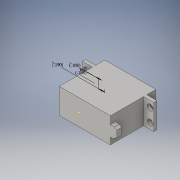
# Autodesk Inventor part: Aidan Sherry Servo motor
Saved by Autodesk Inventor 2016 (Build 200138000, 138)
## iProperties
Created: 2016-10-05
Part Number: Aidan Sherry Servo motor
Material: Generic
Document SubType Name: Modeling
Designer: sherra
Density: 1 g/cm^3
Appearance: Default
Author: sherra
Autodesk Inventor part; units mm, degrees
ref_plane "YZ Plane" through (0, 0, 0) normal (1, 0, 0) x (0, 1, 0)
ref_plane "XZ Plane" through (0, 0, 0) normal (0, 1, 0) x (-1, 0, 0)
ref_plane "XY Plane" through (0, 0, 0) normal (0, 0, 1) x (1, 0, 0)
sketch "Sketch1" plane through (0, 0, 0) normal (0, 0, 1) x (1, 0, 0)
  line L0 (-15.561, 10.0244) -> (24.939, 10.0244)
  line L1 (24.939, 10.0244) -> (24.939, -9.9756)
  line L2 (24.939, -9.9756) -> (-15.561, -9.9756)
  line L3 (-15.561, -9.9756) -> (-15.561, 10.0244)
  point P0 (0, 0)
  dimension "d0" = 20
  dimension "d1" = 40.5
  constraints: 8 end point, 2 parallel, 1 horizontal, 1 perpendicular
  measures "d0" distance between parallel lines of L2 L0
  measures "d1" distance of L0.start L0.end
extrude "Extrusion1" add sketch "Sketch1" along normal blind 36.1
sketch "Sketch2" plane through (24.939, -9.9756, 0) normal (1, 0, 0) x (0, 0, -1)
  line L0 (-36.1, 20) -> (-36.1, 0) projected
  line L1 (-36.1, 13.8904) -> (-32.1201, 13.8904)
  line L2 (-32.1201, 13.8904) -> (-32.1201, 5.486)
  line L3 (-32.1201, 5.486) -> (-36.1, 5.486)
  line L4 (-36.1, 5.486) -> (-36.1, 13.8904)
  point P0 (0, 9.9756)
  constraints: 8 end point, 2 parallel, 1 horizontal, 1 perpendicular, 1 point on line
extrude "Extrusion2" add sketch "Sketch2" along normal blind 5.08
sketch "Sketch3" plane through (24.939, -9.9756, 0) normal (1, 0, 0) x (0, 0, -1)
  line L0 (-36.1, 13.8904) -> (-36.1, 20) projected
  line L1 (-7.2964, 16.9452) -> (-7.2964, 3.5991)
  line L2 (-9.7348, 3.5991) -> (-9.7348, 16.9452)
  line L3 (-9.7348, 16.9452) -> (-9.7348, 20)
  line L4 (0, 20) -> (-36.1, 20) projected
  line L5 (-7.2964, 16.9452) -> (-7.2964, 20)
  line L6 (-7.2964, 3.5991) -> (-7.2964, 0)
  line L7 (0, 0) -> (-36.1, 0) projected
  line L8 (-9.7348, 3.5991) -> (-9.7348, 0)
  point P0 (0, 9.9756)
  constraints: 12 end point, 6 point on line, 2 parallel, 1 vertical
extrude "Extrusion3" add sketch "Sketch3" along normal blind 8.0264
sketch "Sketch4" plane through (-15.561, -9.9756, 0) normal (-1, 0, 0) x (0, 0, 1)
  line L0 (0, 0) -> (7.2964, 0) projected
  line L1 (9.7348, 20) -> (36.1, 20) projected
  line L2 (7.2964, 0) -> (9.7348, 0)
  line L3 (9.7348, 0) -> (9.7348, 20)
  line L4 (9.7348, 20) -> (7.2964, 20)
  line L5 (7.2964, 20) -> (7.2964, 0)
  point P0 (0, 9.9756)
  constraints: 8 end point, 2 parallel, 1 horizontal, 1 perpendicular
extrude "Extrusion4" add sketch "Sketch4" along normal blind 8.0264
sketch "Sketch5" plane through (24.939, -9.9756, 7.2964) normal (0, 0, -1) x (-1, 0, 0)
  line L0 (0, 20) -> (-8.0264, 20) projected
  circle A0 centre (-5.1734, 4.773) radius 2.3347
  line L1 (40.5, 0) -> (48.5264, 0) projected
  line L2 (40.5, 20) -> (48.5264, 20) projected
  circle A1 centre (45.3266, 4.773) radius 2.3347
  circle A2 centre (45.3266, 15.1496) radius 2.3347
  circle A3 centre (-5.1734, 15.1496) radius 2.3347
  point P0 (24.939, 9.9756)
  dimension "d18" = 50.5
  constraints: 4 centre point
  measures "d18" distance of A2.centre A3.centre
hole "Hole1" at (30.1124, -5.2026, 7.2964) at (30.1124, 5.174, 7.2964) at (-20.3876, -5.2026, 7.2964) at (-20.3876, 5.174, 7.2964) direction (0, 0, 1) diameter 4.7625 end through all
sketch "Sketch6" plane through (0, 0, 0) normal (0, 0, -1) x (-1, 0, 0)
  line L0 (15.561, -9.9756) -> (15.561, 10.0244) projected
  line L1 (15.561, 0.0244) -> (-14.839, 0.0244)
  circle A0 centre (-14.839, 0.0244) radius 2.9972
  point P0 (0, 0)
  dimension "d26" = 30.4
  dimension "d27" = 5.9944
  constraints: 2 end point, 1 centre point, 1 coincident, 1 horizontal, 1 midpoint
  measures "d26" distance of L1.start L1.end
  measures "d27" diameter of A0
extrude "Extrusion5" add sketch "Sketch6" along normal blind 5.9944
sketch "Sketch7" plane through (0, 0, 36.1) normal (0, 0, 1) x (1, 0, 0)
  point P0 (0, 0)
sketch "Sketch8" plane through (0, 0, 0) normal (0, 0, -1) x (-1, 0, 0)
  line L0 (15.561, -9.9756) -> (15.561, 10.0244) projected
  circle A0 centre (20.3876, -5.2026) radius 2.3813 projected
  line L1 (15.561, -9.9756) -> (23.5874, -9.9756) projected
  point P0 (0, 0)
  dimension "d30" = 4.8266
  dimension "d31" = 4.7625
  dimension "d33" = 4.773
  measures "d30" distance from line of L0 A0.centre
  measures "d31" diameter of A0
  measures "d33" distance from line of A0.centre L1
body "Solid1"
